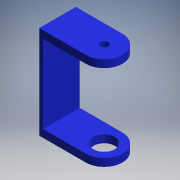
# Autodesk Inventor part: Middle_leg
Saved by Autodesk Inventor 2017 (Build 210142000, 142)
## iProperties
Part Number: Middle_leg
Material: Generic
Document SubType Name: Modeling
Designer: alex-
Appearance: Blue - Wall Paint - Glossy
Author: alex-
Autodesk Inventor part; units mm, degrees
ref_plane "YZ Plane" through (0, 0, 0) normal (1, 0, 0) x (0, 1, 0)
ref_plane "XZ Plane" through (0, 0, 0) normal (0, 1, 0) x (-1, 0, 0)
ref_plane "XY Plane" through (0, 0, 0) normal (0, 0, 1) x (1, 0, 0)
sketch "Sketch3" plane through (0, 0, 0) normal (0, 1, 0) x (-1, 0, 0)
  line L0 (1.25, 12) -> (-1.25, 12)
  line L1 (-1.25, 12) -> (-1.25, -12)
  line L2 (-1.25, -12) -> (1.25, -12)
  line L3 (1.25, -12) -> (1.25, 12)
  point P0 (0, 0)
  point P1 (0, 12)
  point P2 (1.25, 0)
  dimension "d6" = 2.5
  dimension "d7" = 24
  constraints: 8 end point, 2 midpoint, 2 parallel, 1 horizontal, 1 horizontal alignment, 1 perpendicular, 1 vertical alignment
  measures "d6" distance of L0.start L0.end
  measures "d7" distance of L2.end L0.start
extrude "Extrusion3" add sketch "Sketch3" along normal blind 61
sketch "Sketch4" plane through (1.25, 0, 12) normal (1, 0, 0) x (0, 0, -1)
  line L0 (0, 61) -> (24, 61)
  line L1 (24, 61) -> (24, 56)
  line L2 (24, 56) -> (0, 56)
  line L3 (0, 56) -> (0, 61)
  line L4 (0, 5) -> (24, 5)
  line L5 (24, 5) -> (24, 0)
  line L6 (24, 0) -> (0, 0)
  line L7 (0, 0) -> (0, 5)
  line L8 (0, 61) -> (24, 61) projected
  line L9 (0, 0) -> (24, 0) projected
  line L10 (0, 0) -> (0, 61) projected
  point P0 (12, 0)
  point P1 (12, 61)
  point P2 (12, 0)
  point P3 (12, 56)
  point P4 (12, 61)
  point P5 (12, 5)
  point P6 (12, 0)
  point P7 (0, 58.5)
  dimension "d10" = 5
  constraints: 16 end point, 9 midpoint, 4 parallel, 3 point on line, 2 horizontal, 2 perpendicular, 2 vertical alignment, 1 collinear
  measures "d10" distance of L0.end L1.end
extrude "Extrusion4" add sketch "Sketch4" along normal blind 40
fillet "Fillet1" radius 12 2 edges at (41.25, 58.5, 12) (41.25, 58.5, -12)
fillet "Fillet2" radius 12 2 edges at (41.25, 2.5, 12) (41.25, 2.5, -12)
sketch "Sketch6" plane through (0, 61, 0) normal (0, 1, 0) x (1, 0, 0)
  circle A0 centre (29.25, 0) radius 2.5
  arc A1 (29.25, -12) -> (29.25, 12) centre (29.25, 0) ccw projected
  point P0 (0, 0)
  dimension "d16" = 5
  constraints: 1 centre point, 1 concentric
  measures "d16" diameter of A0
extrude "Extrusion5" cut sketch "Sketch6" against normal up to surface (5 mm away)
sketch "Sketch7" plane through (0, 0, 0) normal (0, -1, 0) x (1, 0, 0)
  arc A0 (29.25, -12) -> (29.25, 12) centre (29.25, 0) ccw projected
  circle A1 centre (29.25, 0) radius 7
  point P0 (0, 0)
  dimension "d21" = 14
  constraints: 1 centre point, 1 concentric
  measures "d21" diameter of A1
extrude "Extrusion6" cut sketch "Sketch7" against normal up to surface (5 mm away)
equation "\"d6\" = 0.5 * b_mat_thickness"
equation "\"d7\" = sa_diameter"
equation "\"d8\" = sa_thickness + s_height + s_shaft_height + 3 * b_mat_thickness"
equation "\"d10\" = b_mat_thickness"
equation "\"d14\" = 0.5 * sa_diameter"
equation "\"d15\" = 0.5 * sa_diameter"
equation "\"d21\" = bb_outer_diameter"
equation "\"b_mat_thickness\" = 5"
equation "\"sa_diameter\" = 24"
equation "\"sa_thickness\" = 2"
equation "\"s_height\" = 38"
equation "\"s_shaft_height\" = 6"
equation "\"bb_outer_diameter\" = 14"
body "Solid2"
